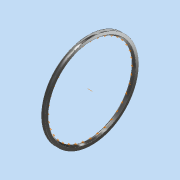
# Autodesk Inventor part: llanta
Saved by Autodesk Inventor 2017 (Build 210142000, 142)
## iProperties
Part Number: llanta
Material: Acero inoxidable
Document SubType Name: Modeling
Designer: Miguel A.
Density: 8 g/cm^3
Appearance: Cromo - Negro Pulido
Author: Miguel A.
Autodesk Inventor part; units mm, degrees
ref_plane "YZ Plane" through (0, 0, 0) normal (1, 0, 0) x (0, 1, 0)
ref_plane "XZ Plane" through (0, 0, 0) normal (0, 1, 0) x (-1, 0, 0)
ref_plane "XY Plane" through (0, 0, 0) normal (0, 0, 1) x (1, 0, 0)
sketch "llanta" plane through (0, 0, 0) normal (0, 0, 1) x (1, 0, 0)
  arc A0 (-5.0239, 188.8921) -> (0, 187.1179) centre (0, 195.1179) ccw
  arc A1 (-16.5, 226.1566) -> (-16.5, 228.1566) centre (-16.5, 227.1566) ccw
  line L0 (-17.5, 228.1566) -> (-16.5, 228.1566)
  arc A2 (-17.5, 228.1566) -> (-18.5, 227.1566) centre (-17.5, 227.1566) ccw
  line L1 (-18.5, 227.1566) -> (-18.5, 202.1566)
  arc A3 (-18.5, 202.1566) -> (-16.6399, 198.2655) centre (-13.5, 202.1566) ccw
  line L2 (-16.6399, 198.2655) -> (-5.0239, 188.8921)
  arc A4 (-5.0239, 188.8921) -> (0, 187.1179) centre (0, 195.1179) ccw
  line L3 (-16.5, 226.1566) -> (-16.5, 202.1566)
  arc A5 (-16.5, 202.1566) -> (-15.3839, 199.822) centre (-13.5, 202.1566) ccw
  line L4 (-15.3839, 199.822) -> (-3.7679, 190.4485)
  arc A6 (-3.7679, 190.4485) -> (0, 189.1179) centre (0, 195.1179) ccw
  line L5 (0, 187.1179) -> (0, 189.1179)
  line L6 (0, 188.1179) -> (0, 205.2521) construction
  line L7 (15.3839, 199.822) -> (3.7679, 190.4485)
  line L8 (16.6399, 198.2655) -> (5.0239, 188.8921)
  arc A7 (0, 189.1179) -> (3.7679, 190.4485) centre (0, 195.1179) ccw
  arc A8 (0, 187.1179) -> (5.0239, 188.8921) centre (0, 195.1179) ccw
  arc A9 (0, 187.1179) -> (5.0239, 188.8921) centre (0, 195.1179) ccw
  arc A10 (15.3839, 199.822) -> (16.5, 202.1566) centre (13.5, 202.1566) ccw
  arc A11 (16.6399, 198.2655) -> (18.5, 202.1566) centre (13.5, 202.1566) ccw
  line L9 (16.5, 226.1566) -> (16.5, 202.1566)
  line L10 (18.5, 227.1566) -> (18.5, 202.1566)
  arc A12 (16.5, 228.1566) -> (16.5, 226.1566) centre (16.5, 227.1566) ccw
  line L11 (17.5, 228.1566) -> (16.5, 228.1566)
  arc A13 (18.5, 227.1566) -> (17.5, 228.1566) centre (17.5, 227.1566) ccw
  point P0 (-50.5, 240.1608)
  dimension "d63" = 2
  dimension "d65" = 25
  dimension "d66" = 5
  dimension "d67" = 8
  dimension "d69" = 2
  measures "d63" distance between parallel lines of L1 L3
  measures "d65" vertical distance of A2.centre A3.centre
  measures "d66" radius of A3
  measures "d67" radius of A4
  measures "d69" diameter of A1
sketch "cubrebola" plane through (0, 0, 0) normal (0, 0, 1) x (1, 0, 0)
  line L0 (-57.0337, 12.8146) -> (-57.0337, 11.8146)
  arc A0 (-57.0337, 11.8146) -> (-53.5337, 8.3146) centre (-53.5337, 11.8146) ccw
  line L1 (-53.5337, 8.3146) -> (-49.0337, 8.3146)
  line L2 (-49.0337, 8.3146) -> (-49.0337, 2.3146)
  line L3 (-57.5337, 13.3146) -> (-65.0337, 13.3146)
  line L4 (-65.0337, 13.3146) -> (-65.0337, 2.3146)
  line L5 (-65.0337, 2.3146) -> (-49.0337, 2.3146)
  line L6 (-53.2763, 2.3146) -> (-52.9205, 2.3146)
  arc A1 (-57.0337, 12.8146) -> (-57.5337, 13.3146) centre (-57.5337, 12.8146) ccw
  line L7 (-65.0337, 6.3146) -> (-49.0337, 6.3146) construction
  point P0 (-57.0337, 13.3146)
  dimension "d26" = 8
  dimension "d27" = 11
  dimension "d28" = 6
  dimension "d29" = 3.5
  dimension "d36" = 8
  dimension "d38" = 0.5
  dimension "d43" = 4
  dimension "d44" = 16
  dimension "d45" = 2
  measures "d26" distance of point (-57.034, 13.315) L3.end
  measures "d27" distance of L3.end L4.end
  measures "d28" distance of L1.end L2.end
  measures "d29" radius of A0
  measures "d36" distance from line of L2 point (-57.034, 13.315)
  measures "d38" radius of A1
  measures "d43" distance between parallel lines of L5 L7
  measures "d44" distance of L7.start L7.end
  measures "d45" distance between parallel lines of L7 L1
sketch "bola eje" plane through (0, 0, 0) normal (0, 0, 1) x (1, 0, 0)
  circle A0 centre (-63.7612, 5.5387) radius 3.5
  dimension "d25" = 3.5
  measures "d25" radius of A0
sketch "eje" plane through (0, 0, 0) normal (0, 0, 1) x (1, 0, 0)
  line L0 (-50.226, 18.6479) -> (-45.226, 18.6479)
  line L1 (-45.226, 18.6479) -> (-40.226, 16.6479)
  line L2 (-48.726, 4.3979) -> (-1.726, 4.3979)
  line L3 (-1.726, 4.3979) -> (-1.726, 16.6479)
  line L4 (-55.726, 11.1479) -> (-55.726, 16.1479)
  line L5 (-55.726, 16.1479) -> (-53.226, 18.6479)
  line L6 (-53.226, 18.6479) -> (-53.226, 27.1479)
  arc A0 (-50.226, 27.1479) -> (-53.226, 27.1479) centre (-51.726, 27.1479) ccw
  line L7 (-50.226, 27.1479) -> (-50.226, 18.6479)
  line L8 (-40.226, 16.6479) -> (-1.726, 16.6479)
  line L9 (-55.726, 11.1479) -> (-52.226, 11.1479)
  arc A1 (-48.726, 7.6479) -> (-52.226, 11.1479) centre (-52.226, 7.6479) ccw
  line L10 (-48.726, 7.6479) -> (-48.726, 4.3979)
  line L11 (-85.079, -1.8521) -> (81.6269, -1.8521) construction
  point P0 (0, 0)
  point P1 (-47.726, 18.6479)
  point P2 (-1.726, 10.5229)
  point P3 (-1.726, -1.8521)
  dimension "d15" = 12.5
  dimension "d47" = 3
  dimension "d48" = 135
  dimension "d49" = 4
  dimension "d50" = 7
  dimension "d51" = 3.5
  dimension "d52" = 5
  dimension "d53" = 12
  dimension "d54" = 2
  dimension "d55" = 5
  dimension "d56" = 5
  dimension "d57" = 12.25
  dimension "d58" = 6.75
  dimension "d59" = 10
  dimension "d62" = 50
  measures "d15" diameter of L2 L11
  measures "d47" distance between parallel lines of L6 L7
  measures "d48" angle of L4 L5
  measures "d49" horizontal distance of L4.end A0.centre
  measures "d50" distance between parallel lines of L10 L4
  measures "d51" radius of A1
  measures "d52" distance of L4.start L4.end
  measures "d54" distance between parallel lines of L8 L0
  measures "d55" distance of L0.start L0.end
  measures "d56" horizontal distance of L1.end L0.end
  measures "d57" distance between parallel lines of L8 L2
  measures "d58" distance between parallel lines of L2 L9
  measures "d62" distance from line of A0.centre L3
derived "madre boceto.ipt"
sketch "Boceto1" plane through (0, 0, 0) normal (0, 0, 1) x (1, 0, 0)
  line L0 (-164.4035, 0) -> (164.4035, 0)
  line L1 (-16.5, 419.0388) -> (-16.5, 421.0388)
  line L2 (16.5, 421.0388) -> (16.5, 419.0388)
  arc A0 (-16.5, 421.0388) -> (16.5, 421.0388) centre (0, 439.8204) ccw
  arc A1 (-16.5, 423.797) -> (16.5, 423.797) centre (0, 439.8204) ccw
  line L3 (16.5, 421.0388) -> (16.5, 423.797)
  line L4 (-16.5, 421.0388) -> (-16.5, 423.797)
  arc A2 (-5.0239, 401.7742) -> (0, 400) centre (0, 408) ccw
  arc A3 (-16.5, 439.0388) -> (-16.5, 441.0388) centre (-16.5, 440.0388) ccw
  line L5 (-17.5, 441.0388) -> (-16.5, 441.0388)
  arc A4 (-17.5, 441.0388) -> (-18.5, 440.0388) centre (-17.5, 440.0388) ccw
  line L6 (-18.5, 440.0388) -> (-18.5, 415.0388)
  arc A5 (-18.5, 415.0388) -> (-16.6399, 411.1476) centre (-13.5, 415.0388) ccw
  line L7 (-16.6399, 411.1476) -> (-5.0239, 401.7742)
  arc A6 (-5.0239, 401.7742) -> (0, 400) centre (0, 408) ccw
  line L8 (-16.5, 439.0388) -> (-16.5, 415.0388)
  arc A7 (-16.5, 415.0388) -> (-15.3839, 412.7041) centre (-13.5, 415.0388) ccw
  line L9 (-15.3839, 412.7041) -> (-3.7679, 403.3306)
  arc A8 (-3.7679, 403.3306) -> (0, 402) centre (0, 408) ccw
  line L10 (0, 400) -> (0, 402)
  line L11 (0, 401) -> (0, 418.1342) construction
  line L12 (15.3839, 412.7041) -> (3.7679, 403.3306)
  line L13 (16.6399, 411.1476) -> (5.0239, 401.7742)
  arc A9 (0, 402) -> (3.7679, 403.3306) centre (0, 408) ccw
  arc A10 (0, 400) -> (5.0239, 401.7742) centre (0, 408) ccw
  arc A11 (0, 400) -> (5.0239, 401.7742) centre (0, 408) ccw
  arc A12 (15.3839, 412.7041) -> (16.5, 415.0388) centre (13.5, 415.0388) ccw
  arc A13 (16.6399, 411.1476) -> (18.5, 415.0388) centre (13.5, 415.0388) ccw
  line L14 (16.5, 439.0388) -> (16.5, 415.0388)
  line L15 (18.5, 440.0388) -> (18.5, 415.0388)
  arc A14 (16.5, 441.0388) -> (16.5, 439.0388) centre (16.5, 440.0388) ccw
  line L16 (17.5, 441.0388) -> (16.5, 441.0388)
  arc A15 (18.5, 440.0388) -> (17.5, 441.0388) centre (17.5, 440.0388) ccw
  point P0 (0, 0)
  point P1 (0, 0)
  dimension "d14" = 2
  dimension "d1" = 400
  dimension "d17" = 25
  dimension "d18" = 20
  dimension "d19" = 20
  dimension "d20" = 2
  constraints: 10 end point, 4 point on circle, 2 centre point, 2 vertical, 1 coincident, 1 horizontal, 1 midpoint, 1 parallel, 8 other
  measures "d17" radius of A0
  measures "d20" radial gap between concentric circles of A1 A0
revolve "Revolución1" add sketch "Boceto1" angle 360 about axis through (-164.4035, 0, 0) along (1, 0, 0) contours L8 A7 L9 A8 L10 A2 L7 A5 L6 A4 L5 A3 L4 L1 | L4 A1 L3 A0 | L3 L14 A14 L16 A15 L15 A13 L13 A10 L10 A9 L12 A12 L2
sketch "Boceto4" plane through (0, 0, 0) normal (0, 1, 0) x (-1, 0, 0)
  line L0 (0, 412.4988) -> (0, 380.1038)
  line L1 (0, 422) -> (6, 422)
  line L2 (6, 422) -> (6, 413)
  line L3 (6, 413) -> (2, 404)
  line L4 (2, 404) -> (2, 395)
  line L5 (2, 395) -> (0, 395)
  line L6 (0, 422) -> (0, 395)
  line L7 (5.0239, 401.7742) -> (5.0239, -401.7742) projected
  line L8 (-5.0239, 401.7742) -> (-5.0239, -401.7742) projected
  arc A0 (-5.0239, 401.7742) -> (5.0239, 401.7742) centre (0, 408) ccw projected
  point P0 (0, 0)
  point P1 (0, 396.3013)
  point P2 (0, 400)
  dimension "d21" = 27
  dimension "d22" = 4
  dimension "d23" = 6
  dimension "d24" = 9
  dimension "d30" = 9
  dimension "d31" = 5
  constraints: 14 end point, 2 perpendicular, 2 point on line, 1 collinear, 1 horizontal, 1 midpoint, 1 parallel, 1 point on circle, 1 vertical, 1 vertical alignment
  measures "d21" distance between parallel lines of L5 L1
  measures "d22" diameter of L4 L0
  measures "d23" distance between parallel lines of L6 L2
  measures "d24" distance of L1.end L2.end
  measures "d30" distance of L3.end L4.end
  measures "d31" distance edge to line of A0 L5
revolve "Revolución5" cut sketch "Boceto4" angle 360 about axis through (0, 0, 412.4988) along (0, 0, -1)
chamfer "Chaflán1" distance 1.5 angle 45 2 edges at (-0.3421, -1.9705, 402.0049) (0.438, 1.9514, 402.0113)
pattern_circular "Patrón circular2" count 36 over 360 about axis through (-16.6399, 0, 0) along (1, 0, 0) of "Revolución5"
equation "\"d18\" = d19"
equation "\"d20\" = d14"
